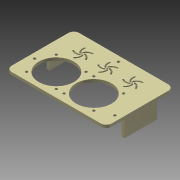
# Autodesk Inventor part: Tapa carcasa SAV
Saved by Autodesk Inventor 2014 (Build 180170000, 170)
## iProperties
Created: 2014-09-11
Part Number: Tapa carcasa SAV
Material: Nylon, molybdenum disulphide
Document SubType Name: Modeling
Designer: Rubén
Density: 1.13 g/cm^3
Appearance: Nylon 6
Mass: 26.3943 g
Surface Area: 167.072 cm^2
Volume: 23.3578 cm^3
Author: Rubén
Autodesk Inventor part; units mm, degrees
ref_plane "YZ Plane" through (0, 0, 0) normal (1, 0, 0) x (0, 1, 0)
ref_plane "XZ Plane" through (0, 0, 0) normal (0, 1, 0) x (-1, 0, 0)
ref_plane "XY Plane" through (0, 0, 0) normal (0, 0, 1) x (1, 0, 0)
sketch "Sketch1" plane through (0, 0, 0) normal (0, 1, 0) x (-1, 0, 0)
  line L0 (6, 0) -> (101.7, 0)
  line L1 (107.7, 6) -> (107.7, 66.77)
  line L2 (101.7, 72.77) -> (6, 72.77)
  line L3 (0, 66.77) -> (0, 6)
  line L4 (6.59, 3) -> (101.11, 3) construction
  line L5 (104.7, 6.59) -> (104.7, 66.18) construction
  line L6 (101.11, 69.77) -> (6.59, 69.77) construction
  line L7 (3, 66.18) -> (3, 6.59) construction
  arc A0 (6.59, 69.77) -> (3, 66.18) centre (6.59, 66.18) ccw construction
  arc A1 (104.7, 66.18) -> (101.11, 69.77) centre (101.11, 66.18) ccw construction
  arc A2 (101.11, 3) -> (104.7, 6.59) centre (101.11, 6.59) ccw construction
  arc A3 (3, 6.59) -> (6.59, 3) centre (6.59, 6.59) ccw construction
  arc A4 (0, 6) -> (6, 0) centre (6, 6) ccw
  arc A5 (101.7, 0) -> (107.7, 6) centre (101.7, 6) ccw
  arc A6 (107.7, 66.77) -> (101.7, 72.77) centre (101.7, 66.77) ccw
  arc A7 (6, 72.77) -> (0, 66.77) centre (6, 66.77) ccw
  circle A8 centre (53.85, 5.8) radius 1.475
  circle A9 centre (5.8, 57.685) radius 1.475
  circle A10 centre (101.9, 47.885) radius 1.475
  line L8 (61.1, 41.9) -> (61.1, 62.5) construction
  line L9 (61.1, 41.9) -> (97.35, 41.9) construction
  line L10 (61.1, 41.9) -> (24.85, 41.9) construction
  line L11 (24.85, 41.9) -> (24.85, 62.5) construction
  line L12 (24.85, 62.5) -> (97.35, 62.5) construction
  line L13 (97.35, 62.5) -> (97.35, 41.9) construction
  line L14 (61.8884, 68.7185) -> (93.8884, 68.7185) construction
  line L15 (98.0634, 64.5435) -> (98.0634, 32.5435) construction
  line L16 (93.8884, 28.3685) -> (61.8884, 28.3685) construction
  line L17 (57.7134, 32.5435) -> (57.7134, 64.5435) construction
  line L18 (53.5384, 68.7185) -> (21.5384, 68.7185) construction
  line L19 (17.3634, 64.5435) -> (17.3634, 32.5435) construction
  line L20 (21.5384, 28.3685) -> (53.5384, 28.3685) construction
  circle A11 centre (21.538, 32.544) radius 1.4
  arc A12 (21.5384, 68.7185) -> (17.3634, 64.5435) centre (21.5384, 64.5435) ccw construction
  arc A13 (17.3634, 32.5435) -> (21.5384, 28.3685) centre (21.5384, 32.5435) ccw construction
  arc A14 (53.5384, 28.3685) -> (57.7134, 32.5435) centre (53.5384, 32.5435) ccw construction
  arc A15 (57.7134, 32.5435) -> (61.8884, 28.3685) centre (61.8884, 32.5435) ccw construction
  arc A16 (93.8884, 28.3685) -> (98.0634, 32.5435) centre (93.8884, 32.5435) ccw construction
  arc A17 (98.0634, 64.5435) -> (93.8884, 68.7185) centre (93.8884, 64.5435) ccw construction
  arc A18 (57.7134, 64.5435) -> (53.5384, 68.7185) centre (53.5384, 64.5435) ccw construction
  arc A19 (61.8884, 68.7185) -> (57.7134, 64.5435) centre (61.8884, 64.5435) ccw construction
  circle A20 centre (21.5384, 64.5435) radius 1.4
  circle A21 centre (61.8884, 64.5435) radius 1.4
  circle A22 centre (53.5384, 64.5435) radius 1.4
  circle A23 centre (93.8884, 64.5435) radius 1.4
  circle A24 centre (61.8884, 32.5435) radius 1.4
  circle A25 centre (53.5384, 32.5435) radius 1.4
  circle A26 centre (93.8884, 32.5435) radius 1.4
  circle A27 centre (37.5384, 48.5435) radius 19
  circle A28 centre (77.8884, 48.5435) radius 19
  circle A29 centre (53.85, 18) radius 0.75
  arc A30 (58.578, 10.8917) -> (56.37, 18.5404) centre (50.85, 12.8038) ccw
  arc A31 (57.122, 11.2519) -> (55.33, 17.4596) centre (50.85, 12.8038) ccw
  arc A32 (57.122, 11.2519) -> (58.578, 10.8917) centre (57.85, 11.0718) ccw
  arc A33 (56.37, 18.5404) -> (55.33, 17.4596) centre (55.85, 18) ccw
  circle A34 centre (80.75, 18) radius 0.75
  arc A35 (85.478, 10.8917) -> (83.27, 18.5404) centre (77.75, 12.8038) ccw
  arc A36 (84.022, 11.2519) -> (82.23, 17.4596) centre (77.75, 12.8038) ccw
  arc A37 (84.022, 11.2519) -> (85.478, 10.8917) centre (84.75, 11.0718) ccw
  arc A38 (83.27, 18.5404) -> (82.23, 17.4596) centre (82.75, 18) ccw
  arc A39 (88.9715, 20.3) -> (81.0148, 20.5637) centre (84.7648, 13.5411) ccw
  arc A40 (88.1789, 19.0266) -> (81.7213, 19.2405) centre (84.7648, 13.5411) ccw
  arc A41 (81.0148, 20.5637) -> (81.7213, 19.2405) centre (81.368, 19.9021) ccw
  arc A42 (88.1789, 19.0266) -> (88.9715, 20.3) centre (88.5752, 19.6633) ccw
  arc A43 (81.1031, 26.5298) -> (78.3936, 19.044) centre (86.2313, 20.4404) ccw
  arc A44 (82.0693, 25.3825) -> (79.8703, 19.3071) centre (86.2313, 20.4404) ccw
  arc A45 (78.3936, 19.044) -> (79.8703, 19.3071) centre (79.132, 19.1756) ccw
  arc A46 (82.0693, 25.3825) -> (81.1031, 26.5298) centre (81.5862, 25.9562) ccw
  arc A47 (72.7468, 20.9717) -> (79.0289, 16.0815) centre (80.1228, 23.9671) ccw
  arc A48 (74.1365, 21.5361) -> (79.235, 17.5673) centre (80.1228, 23.9671) ccw
  arc A49 (79.0289, 16.0815) -> (79.235, 17.5673) centre (79.132, 16.8244) ccw
  arc A50 (74.1365, 21.5361) -> (72.7468, 20.9717) centre (73.4416, 21.2539) ccw
  arc A51 (75.4506, 11.3068) -> (82.0427, 15.7703) centre (74.8811, 19.2475) ccw
  arc A52 (75.3433, 12.8029) -> (80.6934, 16.4255) centre (74.8811, 19.2475) ccw
  arc A53 (82.0427, 15.7703) -> (80.6934, 16.4255) centre (81.368, 16.0979) ccw
  arc A54 (75.3433, 12.8029) -> (75.4506, 11.3068) centre (75.397, 12.0548) ccw
  circle A55 centre (26.95, 18) radius 0.75
  arc A56 (31.678, 10.8917) -> (29.47, 18.5404) centre (23.95, 12.8038) ccw
  arc A57 (30.222, 11.2519) -> (28.43, 17.4596) centre (23.95, 12.8038) ccw
  arc A58 (30.222, 11.2519) -> (31.678, 10.8917) centre (30.95, 11.0718) ccw
  arc A59 (29.47, 18.5404) -> (28.43, 17.4596) centre (28.95, 18) ccw
  arc A60 (35.1715, 20.3) -> (27.2148, 20.5637) centre (30.9648, 13.5411) ccw
  arc A61 (34.3789, 19.0266) -> (27.9213, 19.2405) centre (30.9648, 13.5411) ccw
  arc A62 (27.2148, 20.5637) -> (27.9213, 19.2405) centre (27.568, 19.9021) ccw
  arc A63 (34.3789, 19.0266) -> (35.1715, 20.3) centre (34.7752, 19.6633) ccw
  arc A64 (27.3031, 26.5298) -> (24.5936, 19.044) centre (32.4313, 20.4404) ccw
  arc A65 (28.2693, 25.3825) -> (26.0703, 19.3071) centre (32.4313, 20.4404) ccw
  arc A66 (24.5936, 19.044) -> (26.0703, 19.3071) centre (25.332, 19.1756) ccw
  arc A67 (28.2693, 25.3825) -> (27.3031, 26.5298) centre (27.7862, 25.9562) ccw
  arc A68 (18.9468, 20.9717) -> (25.2289, 16.0815) centre (26.3228, 23.9671) ccw
  arc A69 (20.3365, 21.5361) -> (25.435, 17.5673) centre (26.3228, 23.9671) ccw
  arc A70 (25.2289, 16.0815) -> (25.435, 17.5673) centre (25.332, 16.8244) ccw
  arc A71 (20.3365, 21.5361) -> (18.9468, 20.9717) centre (19.6416, 21.2539) ccw
  arc A72 (21.6506, 11.3068) -> (28.2427, 15.7703) centre (21.0811, 19.2475) ccw
  arc A73 (21.5433, 12.8029) -> (26.8934, 16.4255) centre (21.0811, 19.2475) ccw
  arc A74 (28.2427, 15.7703) -> (26.8934, 16.4255) centre (27.568, 16.0979) ccw
  arc A75 (21.5433, 12.8029) -> (21.6506, 11.3068) centre (21.597, 12.0548) ccw
  circle A76 centre (53.85, 18) radius 0.75
  arc A77 (58.578, 10.8917) -> (56.37, 18.5404) centre (50.85, 12.8038) ccw
  arc A78 (57.122, 11.2519) -> (55.33, 17.4596) centre (50.85, 12.8038) ccw
  arc A79 (57.122, 11.2519) -> (58.578, 10.8917) centre (57.85, 11.0718) ccw
  arc A80 (56.37, 18.5404) -> (55.33, 17.4596) centre (55.85, 18) ccw
  arc A81 (62.0715, 20.3) -> (54.1148, 20.5637) centre (57.8648, 13.5411) ccw
  arc A82 (61.2789, 19.0266) -> (54.8213, 19.2405) centre (57.8648, 13.5411) ccw
  arc A83 (54.1148, 20.5637) -> (54.8213, 19.2405) centre (54.468, 19.9021) ccw
  arc A84 (61.2789, 19.0266) -> (62.0715, 20.3) centre (61.6752, 19.6633) ccw
  arc A85 (54.2031, 26.5298) -> (51.4936, 19.044) centre (59.3313, 20.4404) ccw
  arc A86 (55.1693, 25.3825) -> (52.9703, 19.3071) centre (59.3313, 20.4404) ccw
  arc A87 (51.4936, 19.044) -> (52.9703, 19.3071) centre (52.232, 19.1756) ccw
  arc A88 (55.1693, 25.3825) -> (54.2031, 26.5298) centre (54.6862, 25.9562) ccw
  arc A89 (45.8468, 20.9717) -> (52.1289, 16.0815) centre (53.2228, 23.9671) ccw
  arc A90 (47.2365, 21.5361) -> (52.335, 17.5673) centre (53.2228, 23.9671) ccw
  arc A91 (52.1289, 16.0815) -> (52.335, 17.5673) centre (52.232, 16.8244) ccw
  arc A92 (47.2365, 21.5361) -> (45.8468, 20.9717) centre (46.5416, 21.2539) ccw
  arc A93 (48.5506, 11.3068) -> (55.1427, 15.7703) centre (47.9811, 19.2475) ccw
  arc A94 (48.4433, 12.8029) -> (53.7934, 16.4255) centre (47.9811, 19.2475) ccw
  arc A95 (55.1427, 15.7703) -> (53.7934, 16.4255) centre (54.468, 16.0979) ccw
  arc A96 (48.4433, 12.8029) -> (48.5506, 11.3068) centre (48.497, 12.0548) ccw
  point P0 (0, 0)
  point P1 (107.7, 0)
  point P2 (107.7, 72.77)
  point P3 (3, 3)
  point P4 (104.7, 3)
  point P5 (104.7, 69.77)
  point P6 (3, 69.77)
  point P7 (57.7134, 68.7185)
  point P8 (98.0634, 28.3685)
  point P9 (98.0634, 68.7185)
  point P10 (57.7134, 28.3685)
  point P11 (17.3634, 68.7185)
  point P12 (17.3634, 28.3685)
  dimension "d0" = 107.7
  dimension "d1" = 72.77
  dimension "d2" = 101.7
  dimension "d3" = 66.77
  dimension "d4" = 101.7
  dimension "d5" = 3.59
  dimension "d6" = 3.59
  dimension "d7" = 6
  dimension "d8" = 2.95
  dimension "d9" = 2.95
  dimension "d10" = 2.95
  dimension "d11" = 3
  dimension "d12" = 3
  dimension "d13" = 5.8
  dimension "d14" = 24.885
  dimension "d15" = 53.85
  dimension "d16" = 66.97
  dimension "d17" = 101.9
  dimension "d18" = 15.085
  dimension "d21" = 36.25
  dimension "d22" = 36.25
  dimension "d23" = 20.6
  dimension "d24" = 40.35
  dimension "d25" = 40.35
  dimension "d26" = 40.35
  dimension "d27" = 40.35
  dimension "d28" = 40.35
  dimension "d29" = 2.8
  dimension "d30" = 4.175
  dimension "d31" = 2.8
  dimension "d32" = 2.8
  dimension "d33" = 2.8
  dimension "d34" = 2.8
  dimension "d35" = 2.8
  dimension "d36" = 2.8
  dimension "d37" = 2.8
  dimension "d40" = 38
  dimension "d41" = 38
  dimension "d71" = 26.9
  dimension "d74" = 26.9
  constraints: 160 point on circle, 97 centre point, 42 end point, 36 tangent, 30 point on line, 12 equal radius, 11 perpendicular, 7 coincident, 5 equal length, 4 horizontal, 1 midpoint, 139 other
  measures "d0" distance of point (0, 0) point (107.7, 0)
  measures "d1" distance of point (107.7, 0) point (107.7, 72.77)
  measures "d2" distance of point (3, 3) point (104.7, 3)
  measures "d3" distance of point (104.7, 3) point (104.7, 69.77)
  measures "d4" distance of point (104.7, 69.77) point (3, 69.77)
  measures "d5" radius of A0
  measures "d6" radius of A1
  measures "d7" radius of A4
  measures "d8" diameter of A8
  measures "d9" diameter of A9
  measures "d10" diameter of A10
  measures "d11" distance between parallel lines of L1 L5
  measures "d12" distance between parallel lines of L2 L6
  measures "d13" distance from line of A10.centre L1
  measures "d14" distance from line of A10.centre L2
  measures "d15" distance from line of A8.centre L1
  measures "d16" distance from line of A8.centre L2
  measures "d17" distance from line of A9.centre L1
  measures "d18" distance from line of A9.centre L2
  measures "d21" distance of L8.start L9.end
  measures "d22" distance of L8.start L10.end
  measures "d23" distance of L10.end L11.end
  measures "d24" distance of point (98.063, 28.369) point (57.713, 28.369)
  measures "d25" distance of point (98.063, 68.719) point (98.063, 28.369)
  measures "d26" distance of point (57.713, 68.719) point (17.363, 68.719)
  measures "d27" distance of point (17.363, 68.719) point (17.363, 28.369)
  measures "d28" distance of point (17.363, 28.369) point (57.713, 28.369)
  measures "d29" diameter of A11
  measures "d30" radius of A12
  measures "d31" diameter of A20
  measures "d32" diameter of A21
  measures "d33" diameter of A22
  measures "d34" diameter of A23
  measures "d35" diameter of A24
  measures "d36" diameter of A25
  measures "d37" diameter of A26
  measures "d40" diameter of A27
  measures "d41" diameter of A28
  measures "d71" distance of point (59.331, 20.44) A43.centre
  measures "d74" distance of point (59.331, 20.44) A64.centre
extrude "Extrusion3" add sketch "Sketch1" along normal blind 3
sketch "Sketch2" plane through (0, 0, 0) normal (0, -1, 0) x (1, 0, 0)
  line L0 (-6, 72.77) -> (-101.7, 72.77) projected
  line L1 (-107.7, 66.77) -> (-107.7, 6) projected
  line L2 (-107.7, 10.685) -> (-104.7, 10.685)
  line L3 (-107.7, 28.985) -> (-104.7, 28.985)
  line L4 (-104.7, 28.985) -> (-104.7, 10.685)
  line L5 (-107.7, 28.985) -> (-107.7, 10.685)
  point P0 (0, 0)
  dimension "d44" = 3
  dimension "d45" = 43.785
  dimension "d46" = 62.085
  constraints: 8 end point, 2 perpendicular, 2 point on line, 1 collinear, 1 parallel
  measures "d44" distance of L2.start L2.end
  measures "d45" distance between parallel lines of L0 L3
  measures "d46" distance between parallel lines of L0 L2
extrude "Extrusion4" add sketch "Sketch2" along normal blind 19
sketch "Sketch3" plane through (0, 0, 0) normal (0, -1, 0) x (1, 0, 0)
  line L0 (0, 6) -> (0, 66.77) projected
  line L1 (-107.7, 66.77) -> (-107.7, 28.985) projected
  line L2 (0, 17.985) -> (-3, 17.985)
  line L3 (0, 53.085) -> (-3, 53.085)
  line L4 (-3, 53.085) -> (-3, 17.985)
  line L5 (0, 17.985) -> (0, 53.085)
  point P0 (0, 0)
  dimension "d49" = 3
  dimension "d50" = 3
  constraints: 8 end point, 2 point on line, 1 collinear, 1 parallel, 1 perpendicular
  measures "d49" distance of L2.start L2.end
  measures "d50" distance of L3.start L3.end
extrude "Extrusion5" add sketch "Sketch3" along normal blind 17.616
body "Solid3"
